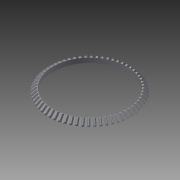
# Autodesk Inventor part: Beveled_Ring
Saved by Autodesk Inventor 2015 (Build 190159000, 159)
## iProperties
Created: 2016-02-12
Part Number: Beveled_Ring
Material: Generic
Document SubType Name: Modeling
Designer: david_000
Density: 1 g/cm^3
Appearance: Default
Author: david_000
Autodesk Inventor part; units mm, degrees
ref_plane "YZ Plane" through (0, 0, 0) normal (1, 0, 0) x (0, 1, 0)
ref_plane "XZ Plane" through (0, 0, 0) normal (0, 1, 0) x (-1, 0, 0)
ref_plane "XY Plane" through (0, 0, 0) normal (0, 0, 1) x (1, 0, 0)
sketch "Sketch15" plane through (0, 0, 0) normal (0, 1, 0) x (-1, 0, 0)
  line L0 (0, 0) -> (-171.45, 0)
  line L1 (0, 0) -> (-171.45, 0) construction
  line L2 (0, 0) -> (-170.5108, 17.9214) construction
  line L3 (0, 0) -> (-171.45, 0) construction
  line L4 (-171.45, 0) -> (-171.1491, 10.1532)
  line L5 (-171.1491, 10.1532) -> (-170.5108, 17.9214)
  line L6 (-170.5108, 17.9214) -> (0, 0)
  dimension "d52" = 171.45
  dimension "d54" = 6
  constraints: 14 end point, 3 coincident, 1 horizontal
  measures "d52" distance of L0.start L0.end
  measures "d54" angle of L2 L3
extrude "Extrusion12" add sketch "Sketch15" along normal blind 19.05
chamfer "Chamfer1" distance 19.05 angle 45 2 edges at (171.2995, 0, 5.0766) (170.8299, 0, 14.0373)
pattern_circular "Circular Pattern5" count 60 over 360 about axis through (0, 0, 0) along (0, 1, 0) of "Extrusion12", "Chamfer1"
sketch "Sketch16" plane through (113.2491, 0, -101.9699) normal (0.5392681, -0.7071068, -0.4573728) x (0.5255981, 0.7069516, -0.4732506)
  line L0 (0.0024, -0.0001) -> (26.9467, 0)
  line L1 (26.9467, 0) -> (26.7339, 10.1555)
  line L2 (26.7339, 10.1555) -> (-0.1905, 9.0923)
  line L3 (26.7339, 10.1555) -> (-0.1905, 9.0923) projected
  line L4 (-0.1905, 9.0923) -> (0.0024, -0.0001)
  point P0 (-107.7808, 2.2566)
  constraints: 8 end point, 1 collinear
extrude "Extrusion13" add sketch "Sketch16" along normal blind 6.35 draft -23.6
sketch "Sketch17" plane through (0, 0, 0) normal (0, -1, 0) x (1, 0, 0)
  circle A0 centre (0, 0) radius 152.4
  dimension "d65" = 304.8
  constraints: 1 centre point, 1 coincident
  measures "d65" diameter of A0
extrude "Extrusion14" cut sketch "Sketch17" against normal up to next
pattern_circular "Circular Pattern6" count 60 over 360 about axis through (0, 0, 0) along (0, 1, 0) of "Extrusion13"
body "Solid5"
